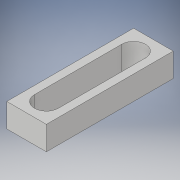
# Autodesk Inventor part: creat10
Saved by Autodesk Inventor 2019 (Build 230136000, 136)
## iProperties
Created: 2021-11-15
Part Number: creat10
Material: 一般
Document SubType Name: Modeling
Designer: yuta
Density: 1 g/cm^3
Appearance: 既定
Author: yuta
Autodesk Inventor part; units mm, degrees
ref_plane "YZ Plane" through (0, 0, 0) normal (1, 0, 0) x (0, 1, 0)
ref_plane "XZ Plane" through (0, 0, 0) normal (0, 1, 0) x (-1, 0, 0)
ref_plane "XY Plane" through (0, 0, 0) normal (0, 0, 1) x (1, 0, 0)
sketch "スケッチ1" plane through (0, 0, 0) normal (0, 0, 1) x (1, 0, 0)
  point P0 (0, 0)
sketch "スケッチ2" plane through (0, 0, 0) normal (0, 1, 0) x (-1, 0, 0)
  line L0 (2.109, 9.3486) -> (-2.891, 9.3486)
  line L1 (-2.891, 9.3486) -> (-2.891, -6.6514)
  line L2 (-2.891, -6.6514) -> (2.109, -6.6514)
  line L3 (2.109, -6.6514) -> (2.109, 9.3486)
  point P0 (0, 0)
  dimension "d0" = 5
  dimension "d1" = 16
  constraints: 8 end point, 2 parallel, 1 horizontal, 1 perpendicular
  measures "d0" distance of L2.end L1.end
  measures "d1" distance of L2.end L0.start
extrude "押し出し1" add sketch "スケッチ2" along normal blind 3
sketch "スケッチ3" plane through (0, 3, 0) normal (0, 1, 0) x (1, 0, 0)
  line L0 (0.391, -6.8486) -> (0.391, 4.1514) construction
  line L1 (1.891, -6.8486) -> (1.891, 4.1514)
  line L2 (-1.109, 4.1514) -> (-1.109, -6.8486)
  arc A0 (-1.109, -6.8486) -> (1.891, -6.8486) centre (0.391, -6.8486) ccw
  arc A1 (1.891, 4.1514) -> (-1.109, 4.1514) centre (0.391, 4.1514) ccw
  line L3 (-2.109, 6.6514) -> (-2.109, -9.3486) projected
  line L4 (-2.109, -9.3486) -> (2.891, -9.3486) projected
  point P0 (0, 0)
  point P1 (0.391, -1.3486)
  dimension "d4" = 11
  dimension "d5" = 3
  dimension "d6" = 1
  dimension "d7" = 2.5
  constraints: 8 end point, 4 point on circle, 4 tangent, 2 centre point, 1 midpoint, 1 parallel, 1 vertical
  measures "d4" distance of L0.start L0.end
  measures "d5" diameter of A1
  measures "d6" distance between parallel lines of L3 L2
  measures "d7" distance from line of L4 L0.start
extrude "押し出し2" cut sketch "スケッチ3" against normal blind 3
